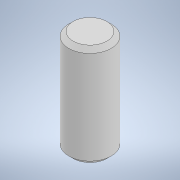
# Autodesk Inventor part: 78. Стопорный палец
Saved by Autodesk Inventor 2021 (Build 250183000, 183)
## iProperties
Created: 2021-03-18
Part Number: 78. Стопорный палец
Material: Типовые
Document SubType Name: Modeling
Designer: Данил
Density: 1 g/cm^3
Appearance: По умолчанию
Author: Данил
Autodesk Inventor part; units mm, degrees
ref_plane "YZ Plane" through (0, 0, 0) normal (1, 0, 0) x (0, 1, 0)
ref_plane "XZ Plane" through (0, 0, 0) normal (0, 1, 0) x (-1, 0, 0)
ref_plane "XY Plane" through (0, 0, 0) normal (0, 0, 1) x (1, 0, 0)
sketch "Эскиз1" plane through (0, 0, 0) normal (0, 0, 1) x (1, 0, 0)
  line L0 (0, 6) -> (0, -6)
  line L1 (0, 6) -> (2, 6)
  line L2 (2.5, 5.5) -> (2.5, -5.5)
  line L3 (2, -6) -> (0, -6)
  line L4 (0, -6) -> (0, 6)
  line L5 (2.5, -5.5) -> (2, -6)
  line L6 (2.5, 5.5) -> (2, 6)
  point P0 (0, 0)
  point P1 (0, 0)
  point P2 (2.5, -6)
  point P3 (2.5, 6)
  dimension "d0" = 12
  dimension "d1" = 5
  dimension "d2" = 0.5
  dimension "d3" = 45
  dimension "d4" = 0.5
  dimension "d5" = 45
  constraints: 14 end point, 4 point on line, 2 parallel, 1 coincident, 1 horizontal, 1 midpoint, 1 perpendicular, 1 vertical
  measures "d0" distance of L0.start L0.end
  measures "d1" diameter of L2 L0
  measures "d2" distance of L2.end point (2.5, -6)
  measures "d3" angle of L2 L5
  measures "d4" distance of L2.start point (2.5, 6)
  measures "d5" angle of L2 L6
revolve "Вращение1" add sketch "Эскиз1" angle 360 about axis through (0, 6, 0) along (0, -1, 0)
equation "\"d4\" = d2"
equation "\"d5\" = d3"
